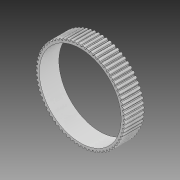
# Autodesk Inventor part: HD_FlexSpline_3m_198_15
Saved by Autodesk Inventor 2020 (Build 240168000, 168)
## iProperties
Created: 2021-04-04
Part Number: HD_FlexSpline_3m_198_15
Material: Generic
Document SubType Name: Modeling
Designer: DDeGo
Density: 1 g/cm^3
Appearance: Default
Author: DDeGo
Autodesk Inventor part; units mm, degrees
ref_plane "YZ Plane" through (0, 0, 0) normal (1, 0, 0) x (0, 1, 0)
ref_plane "XZ Plane" through (0, 0, 0) normal (0, 1, 0) x (-1, 0, 0)
ref_plane "XY Plane" through (0, 0, 0) normal (0, 0, 1) x (1, 0, 0)
sketch "Sketch1" plane through (0, 0, 0) normal (0, 0, 1) x (1, 0, 0)
  circle A0 centre (0, 0) radius 32.945
  circle A1 centre (0, 0) radius 31.445
  dimension "d0" = 65.89
  dimension "d1" = 1.5
  constraints: 2 centre point, 2 coincident
  measures "d0" diameter of A0
  measures "d1" radial gap between concentric circles of A1 A0
extrude "Extrusion1" add sketch "Sketch1" along normal mid plane 15
sketch "Sketch2" plane through (0, 0, 7.5) normal (0, 0, 1) x (1, 0, 0)
  circle A0 centre (-33.32, 0) radius 0.875
  circle A1 centre (0, 0) radius 34.195 construction
  circle A2 centre (0, 0) radius 32.945 construction
  line L0 (-33.32, 0) -> (0, 0) construction
  dimension "d4" = 1.25
  dimension "d5" = 1.75
  constraints: 2 centre point, 2 end point, 1 coincident, 1 horizontal, 1 tangent
  measures "d4" radial gap between concentric circles of A2 A1
  measures "d5" diameter of A0
extrude "Extrusion2" add sketch "Sketch2" against normal up to surface (15 mm away)
fillet "Fillet1" radius 0.5 4 edges at (-32.9356, -0.7861, 3.75) (-32.9356, -0.7861, -3.75) (-32.9356, 0.7861, 3.75) (-32.9356, 0.7861, -3.75)
pattern_circular "Circular Pattern1" count 69 over 360 about axis through (0, 0, 0) along (0, 0, 1) of "Fillet1", "Extrusion2"
body "Solid1"
